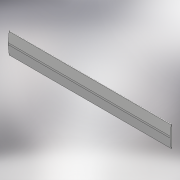
# Autodesk Inventor part: foward_flap
Saved by Autodesk Inventor 2018.2 (Build 222227000, 227)
## iProperties
Created: 2017-12-14
Part Number: foward_flap
Material: 一般
Document SubType Name: Modeling
Designer: kuwano
Density: 1 g/cm^3
Appearance: 既定
Author: kuwano
Autodesk Inventor part; units mm, degrees
ref_plane "YZ Plane" through (0, 0, 0) normal (1, 0, 0) x (0, 1, 0)
ref_plane "XZ Plane" through (0, 0, 0) normal (0, 1, 0) x (-1, 0, 0)
ref_plane "XY Plane" through (0, 0, 0) normal (0, 0, 1) x (1, 0, 0)
sketch "スケッチ1" plane through (0, 0, 0) normal (1, 0, 0) x (0, 1, 0)
  line L0 (10, 100) -> (10, -100)
  line L1 (10, -100) -> (0, 0)
  line L2 (0, 0) -> (10, 100)
  line L3 (-2, 0) -> (12, 0) projected
  point P0 (10, 0)
  dimension "d0" = 200
  dimension "d5" = 10
  constraints: 6 end point, 1 midpoint, 1 point on line, 1 vertical
  measures "d0" distance of L0.start L0.end
  measures "d5" distance of L1.end point (10, 0)
extrude "押し出し1" add sketch "スケッチ1" along normal mid plane 950
fillet "フィレット1" radius 2 2 edges at (0, 10, 100) (0, 10, -100)
fillet "フィレット1" radius 50 1 edges at (0, 0, 0)
